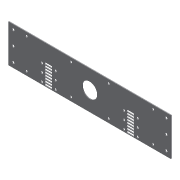
# Autodesk Inventor part: elevbackpltblt
Saved by Autodesk Inventor 2015 SP1 (Build 190203100, 203)
## iProperties
Created: 2015-01-20
Part Number: elevbackpltblt
Material: Generic
Document SubType Name: Modeling
Designer: Owner
Density: 1 g/cm^3
Appearance: Default
Author: Owner
Autodesk Inventor part; units mm, degrees
ref_plane "YZ Plane" through (0, 0, 0) normal (1, 0, 0) x (0, 1, 0)
ref_plane "XZ Plane" through (0, 0, 0) normal (0, 1, 0) x (-1, 0, 0)
ref_plane "XY Plane" through (0, 0, 0) normal (0, 0, 1) x (1, 0, 0)
sketch "Sketch1" plane through (0, 0, 0) normal (0, 0, 1) x (1, 0, 0)
  line L0 (0, 0) -> (436.118, 0)
  line L1 (436.118, 0) -> (436.118, 101.6)
  line L2 (436.118, 101.6) -> (0, 101.6)
  line L3 (0, 101.6) -> (0, 0)
  circle A0 centre (12.7, 88.9) radius 3.3655
  circle A1 centre (12.7, 50.8) radius 3.3655
  circle A2 centre (12.7, 12.7) radius 3.3655
  circle A3 centre (423.418, 88.9) radius 3.3655
  circle A4 centre (423.418, 50.8) radius 3.3655
  circle A5 centre (423.418, 12.7) radius 3.3655
  circle A6 centre (218.059, 50.8) radius 20.32
  dimension "d0" = 436.118
  dimension "d1" = 101.6
  dimension "d2" = 6.731
  dimension "d3" = 12.7
  dimension "d4" = 12.7
  dimension "d7" = 38.1
  dimension "d10" = 410.718
  dimension "d13" = 12.7
  dimension "d24" = 40.64
  dimension "d25" = 50.8
  dimension "d26" = 218.059
  constraints: 8 end point, 7 centre point, 2 horizontal, 2 parallel, 1 perpendicular, 1 vertical, 10 other
  measures "d0" distance of L2.end L1.end
  measures "d1" distance between parallel lines of L0 L2
  measures "d2" diameter of A0
  measures "d3" distance from line of L3 A0.centre
  measures "d4" distance from line of L2 A0.centre
  measures "d7" distance of A0.centre A1.centre
  measures "d10" distance of A0.centre A3.centre
  measures "d13" distance from line of A3.centre L1
  measures "d24" diameter of A6
  measures "d25" distance from line of L2 A6.centre
  measures "d26" distance from line of L3 A6.centre
extrude "Extrusion1" add sketch "Sketch1" along normal blind 2.286
sketch "Sketch2" plane through (0, 0, 2.286) normal (0, 0, 1) x (1, 0, 0)
  line L0 (0, 0) -> (436.118, 0) projected
  line L1 (82.55, 0) -> (133.35, 0)
  line L2 (31.75, 101.6) -> (184.15, 101.6)
  line L3 (133.35, 0) -> (184.15, 101.6)
  line L4 (31.75, 101.6) -> (82.55, 0)
  line L5 (97.1739, 7) -> (117.1739, 7)
  line L6 (117.1739, 7) -> (117.1739, 2)
  line L7 (117.1739, 2) -> (97.1739, 2)
  line L8 (97.1739, 2) -> (97.1739, 7)
  line L9 (133.35, 0) -> (133.35, 62.4863)
  line L10 (97.1739, 14) -> (117.1739, 14)
  line L11 (117.1739, 14) -> (117.1739, 9)
  line L12 (117.1739, 9) -> (97.1739, 9)
  line L13 (97.1739, 9) -> (97.1739, 14)
  line L14 (97.1739, 21) -> (117.1739, 21)
  line L15 (117.1739, 21) -> (117.1739, 16)
  line L16 (117.1739, 16) -> (97.1739, 16)
  line L17 (97.1739, 16) -> (97.1739, 21)
  line L18 (97.1739, 28) -> (117.1739, 28)
  line L19 (117.1739, 28) -> (117.1739, 23)
  line L20 (117.1739, 23) -> (97.1739, 23)
  line L21 (97.1739, 23) -> (97.1739, 28)
  line L22 (97.1739, 35) -> (117.1739, 35)
  line L23 (117.1739, 35) -> (117.1739, 30)
  line L24 (117.1739, 30) -> (97.1739, 30)
  line L25 (97.1739, 30) -> (97.1739, 35)
  line L26 (97.1739, 42) -> (117.1739, 42)
  line L27 (117.1739, 42) -> (117.1739, 37)
  line L28 (117.1739, 37) -> (97.1739, 37)
  line L29 (97.1739, 37) -> (97.1739, 42)
  circle A0 centre (126.2557, 6.2222) radius 3.1623
  circle A1 centre (126.2557, 28) radius 3.1623
  circle A2 centre (126.2557, 49.7778) radius 3.1623
  line L30 (107.95, 0) -> (107.95, -15.6085)
  circle A3 centre (89.6443, 49.7778) radius 3.1623
  circle A4 centre (89.6443, 6.2222) radius 3.1623
  circle A5 centre (89.6443, 28) radius 3.1623
  line L31 (117.1739, 44) -> (97.1739, 44)
  line L32 (97.1739, 44) -> (97.1739, 49)
  line L33 (117.1739, 49) -> (117.1739, 44)
  line L34 (97.1739, 49) -> (117.1739, 49)
  line L35 (117.1739, 51) -> (97.1739, 51)
  line L36 (97.1739, 51) -> (97.1739, 56)
  line L37 (97.1739, 56) -> (117.1739, 56)
  line L38 (117.1739, 56) -> (117.1739, 51)
  circle A6 centre (48.26, 91.44) radius 3.1623
  circle A7 centre (167.64, 91.44) radius 3.1623
  circle A8 centre (48.26, 10.16) radius 3.1623
  circle A9 centre (167.64, 10.16) radius 3.1623
  point P0 (0, 101.6)
  dimension "d37" = 50.8
  dimension "d38" = 152.4
  dimension "d39" = 101.6
  dimension "d40" = 50.8
  dimension "d41" = 20
  dimension "d42" = 5
  dimension "d43" = 2
  dimension "d44" = 7
  dimension "d45" = 6.3246
  dimension "d46" = 6.3246
  dimension "d47" = 6.3246
  dimension "d48" = 14
  dimension "d49" = 56
  dimension "d50" = 6.2222
  dimension "d51" = 6.2222
  dimension "d52" = 28
  dimension "d53" = 6.3246
  dimension "d54" = 6.3246
  dimension "d55" = 34.29
  dimension "d56" = 34.29
  dimension "d57" = 10.16
  dimension "d58" = 10.16
  dimension "d61" = 16.1761
  dimension "d62" = 31.75
  dimension "d112" = 9.0818
  dimension "d113" = 9.0818
  dimension "d114" = 9.0818
  dimension "d115" = 6.3246
  dimension "d116" = 10.16
  dimension "d117" = 34.29
  dimension "d118" = 6.3246
  dimension "d119" = 10.16
  dimension "d120" = 34.29
  constraints: 76 end point, 10 centre point, 4 vertical, 3 parallel, 3 symmetric about line, 2 horizontal, 1 collinear, 1 midpoint, 1 perpendicular, 59 other
  measures "d37" distance of L1.start L1.end
  measures "d38" distance of L2.start L2.end
  measures "d39" distance between parallel lines of L2 L1
  measures "d40" horizontal distance of L2.end L1.end
  measures "d41" distance of L6.end L7.end
  measures "d42" distance between parallel lines of L5 L7
  measures "d43" distance between parallel lines of L1 L7
  measures "d44" distance of L5.start L10.start
  measures "d45" diameter of A0
  measures "d46" diameter of A1
  measures "d47" diameter of A2
  measures "d48" distance of L24.end L31.end
  measures "d49" distance between parallel lines of L1 L37
  measures "d50" distance from line of L37 A2.centre
  measures "d51" distance from line of L1 A0.centre
  measures "d52" distance from line of L1 A1.centre
  measures "d53" diameter of A6
  measures "d54" diameter of A7
  measures "d55" horizontal distance of A7.centre L1.end
  measures "d56" horizontal distance of A6.centre L1.start
  measures "d57" vertical distance of A6.centre L2.start
  measures "d58" vertical distance of A7.centre L2.end
  measures "d61" distance from line of L1.end L6
  measures "d62" distance of L2.start point (0, 101.6)
  measures "d112" distance from line of L38 A2.centre
  measures "d113" distance from line of L23 A1.centre
  measures "d114" distance from line of L11 A0.centre
  measures "d115" diameter of A8
  measures "d116" distance from line of L0 A8.centre
  measures "d117" horizontal distance of A8.centre L1.start
  measures "d118" diameter of A9
  measures "d119" distance from line of L0 A9.centre
  measures "d120" horizontal distance of L1.end A9.centre
extrude "Extrusion2" cut sketch "Sketch2" against normal blind 2.286 contours L5 L6 L7 L8 | L10 L11 L12 L13 | L14 L15 L16 L17 | L18 L19 L20 L21 | L22 L23 L24 L25 | L26 L27 L28 L29 | A0 | A1 | A2 | A3 | A4 | A5 | L31 L32 L34 L33 | L35 L36 L37 L38 | A6 | A7 | A8 | A9
sketch "Sketch3" plane through (0, 0, 2.286) normal (0, 0, 1) x (1, 0, 0)
  circle A0 centre (126.2557, 49.7778) radius 3.1623 projected
  line L0 (117.1739, 56) -> (117.1739, 51) projected
  line L1 (0, 0) -> (436.118, 0) projected
  line L2 (302.768, 0) -> (353.568, 0)
  line L3 (251.968, 101.6) -> (404.368, 101.6)
  line L4 (353.568, 0) -> (404.368, 101.6)
  line L5 (251.968, 101.6) -> (302.768, 0)
  line L6 (317.3919, 7) -> (337.3919, 7)
  line L7 (337.3919, 7) -> (337.3919, 2)
  line L8 (337.3919, 2) -> (317.3919, 2)
  line L9 (317.3919, 2) -> (317.3919, 7)
  line L10 (353.568, 0) -> (353.568, 62.4863)
  line L11 (317.3919, 14) -> (337.3919, 14)
  line L12 (337.3919, 14) -> (337.3919, 9)
  line L13 (337.3919, 9) -> (317.3919, 9)
  line L14 (317.3919, 9) -> (317.3919, 14)
  line L15 (317.3919, 21) -> (337.3919, 21)
  line L16 (337.3919, 21) -> (337.3919, 16)
  line L17 (337.3919, 16) -> (317.3919, 16)
  line L18 (317.3919, 16) -> (317.3919, 21)
  line L19 (317.3919, 28) -> (337.3919, 28)
  line L20 (337.3919, 28) -> (337.3919, 23)
  line L21 (337.3919, 23) -> (317.3919, 23)
  line L22 (317.3919, 23) -> (317.3919, 28)
  line L23 (317.3919, 35) -> (337.3919, 35)
  line L24 (337.3919, 35) -> (337.3919, 30)
  line L25 (337.3919, 30) -> (317.3919, 30)
  line L26 (317.3919, 30) -> (317.3919, 35)
  line L27 (317.3919, 42) -> (337.3919, 42)
  line L28 (337.3919, 42) -> (337.3919, 37)
  line L29 (337.3919, 37) -> (317.3919, 37)
  line L30 (317.3919, 37) -> (317.3919, 42)
  circle A1 centre (346.4737, 6.2222) radius 3.1623
  circle A2 centre (346.4737, 28) radius 3.1623
  circle A3 centre (346.4737, 49.7778) radius 3.1623
  line L31 (328.168, 0) -> (328.168, -15.6085)
  circle A4 centre (309.8623, 49.7778) radius 3.1623
  circle A5 centre (309.8623, 6.2222) radius 3.1623
  circle A6 centre (309.8623, 28) radius 3.1623
  line L32 (337.3919, 44) -> (317.3919, 44)
  line L33 (317.3919, 44) -> (317.3919, 49)
  line L34 (337.3919, 49) -> (337.3919, 44)
  line L35 (317.3919, 49) -> (337.3919, 49)
  line L36 (337.3919, 51) -> (317.3919, 51)
  line L37 (317.3919, 51) -> (317.3919, 56)
  line L38 (317.3919, 56) -> (337.3919, 56)
  line L39 (337.3919, 56) -> (337.3919, 51)
  circle A7 centre (268.478, 91.44) radius 3.1623
  circle A8 centre (387.858, 91.44) radius 3.1623
  circle A9 centre (268.478, 10.16) radius 3.1623
  circle A10 centre (387.858, 10.16) radius 3.1623
  point P0 (436.118, 101.6)
  dimension "d74" = 50.8
  dimension "d75" = 152.4
  dimension "d76" = 101.6
  dimension "d77" = 50.8
  dimension "d78" = 20
  dimension "d79" = 5
  dimension "d80" = 2
  dimension "d81" = 7
  dimension "d82" = 6.3246
  dimension "d83" = 6.3246
  dimension "d84" = 6.3246
  dimension "d85" = 14
  dimension "d86" = 56
  dimension "d87" = 6.2222
  dimension "d88" = 6.2222
  dimension "d89" = 28
  dimension "d90" = 6.3246
  dimension "d91" = 6.3246
  dimension "d92" = 34.29
  dimension "d93" = 34.29
  dimension "d94" = 10.16
  dimension "d95" = 10.16
  dimension "d98" = 16.1761
  dimension "d99" = 31.75
  dimension "d100" = 9.0818
  dimension "d101" = 9.0818
  dimension "d102" = 9.0818
  dimension "d103" = 9.0818
  dimension "d104" = 6.3246
  dimension "d105" = 10.16
  dimension "d106" = 34.29
  dimension "d107" = 6.3246
  dimension "d108" = 10.16
  dimension "d109" = 34.29
  constraints: 76 end point, 10 centre point, 4 vertical, 3 parallel, 3 symmetric about line, 2 horizontal, 1 collinear, 1 midpoint, 1 perpendicular, 59 other
  measures "d74" distance of L2.start L2.end
  measures "d75" distance of L3.start L3.end
  measures "d76" distance between parallel lines of L3 L2
  measures "d77" horizontal distance of L3.end L2.end
  measures "d78" distance of L7.end L8.end
  measures "d79" distance between parallel lines of L6 L8
  measures "d80" distance between parallel lines of L2 L8
  measures "d81" distance of L6.start L11.start
  measures "d82" diameter of A1
  measures "d83" diameter of A2
  measures "d84" diameter of A3
  measures "d85" distance of L25.end L32.end
  measures "d86" distance between parallel lines of L2 L38
  measures "d87" distance from line of L38 A3.centre
  measures "d88" distance from line of L2 A1.centre
  measures "d89" distance from line of L2 A2.centre
  measures "d90" diameter of A7
  measures "d91" diameter of A8
  measures "d92" horizontal distance of A8.centre L2.end
  measures "d93" horizontal distance of A7.centre L2.start
  measures "d94" vertical distance of A7.centre L3.start
  measures "d95" vertical distance of A8.centre L3.end
  measures "d98" distance from line of L2.end L7
  measures "d99" distance of point (436.118, 101.6) L3.end
  measures "d100" distance from line of L39 A3.centre
  measures "d101" distance from line of L0 A0.centre
  measures "d102" distance from line of L20 A2.centre
  measures "d103" distance from line of L12 A1.centre
  measures "d104" diameter of A9
  measures "d105" distance from line of L1 A9.centre
  measures "d106" horizontal distance of L2.start A9.centre
  measures "d107" diameter of A10
  measures "d108" distance from line of L1 A10.centre
  measures "d109" horizontal distance of L2.end A10.centre
extrude "Extrusion3" cut sketch "Sketch3" against normal blind 6.3246 contours L6 L7 L8 L9 | L11 L12 L13 L14 | L15 L16 L17 L18 | L19 L20 L21 L22 | L23 L24 L25 L26 | L27 L28 L29 L30 | A1 | A2 | A3 | A4 | A5 | A6 | L32 L33 L35 L34 | L36 L37 L38 L39 | A7 | A8 | A9 | A10
equation "\"d26\" = 0.5 * d0"
equation "\"d46\" = d45"
equation "\"d47\" = d46"
equation "\"d50\" = 0.111111 * d49"
equation "\"d51\" = d50"
equation "\"d52\" = 0.5 * d49"
equation "\"d56\" = d55"
equation "\"d58\" = d57"
equation "\"d113\" = d112"
equation "\"d114\" = d112"
equation "\"d116\" = d57"
equation "\"d117\" = d56"
equation "\"d119\" = d58"
equation "\"d120\" = d55"
equation "\"d83\" = d82"
equation "\"d84\" = d83"
equation "\"d87\" = 0.111111 * d86"
equation "\"d88\" = d87"
equation "\"d89\" = 0.5 * d86"
equation "\"d93\" = d92"
equation "\"d95\" = d94"
equation "\"d102\" = d100"
equation "\"d103\" = d100"
equation "\"d105\" = d94"
equation "\"d106\" = d93"
equation "\"d108\" = d95"
equation "\"d109\" = d92"
equation "\"d110\" = d83"
body "Solid1"
